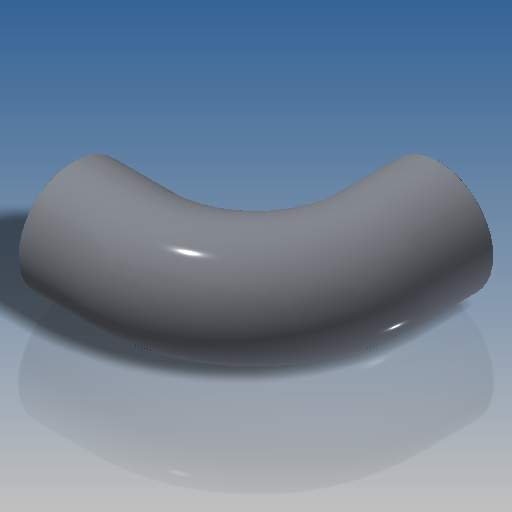
# Autodesk Inventor part: 25214-LtBluishGray
Saved by Autodesk Inventor 2019.4 (Build 234330000, 330)
## iProperties
Created: 2016-10-12
Part Number: 25214-LtBluishGray
Material: ABS Plastic
Document SubType Name: Modeling
Designer: D. Kohfeld
Density: 1.06 g/cm^3
Appearance: LtBluishGray
Mass: 0.6342 g
Surface Area: 8.19784 cm^2
Volume: 0.598302 cm^3
Author: D. Kohfeld
Autodesk Inventor part; units mm, degrees
ref_plane "YZ Plane" through (0, 0, 0) normal (1, 0, 0) x (0, 1, 0)
ref_plane "XZ Plane" through (0, 0, 0) normal (0, 1, 0) x (-1, 0, 0)
sketch "Sketch2" plane through (0, 0, 0) normal (0, 1, 0) x (-1, 0, 0)
  line L0 (0, -12) -> (0, -8)
  arc A0 (8, 0) -> (0, -8) centre (8, -8) ccw
  line L1 (8, 0) -> (12, 0)
  point P0 (0, 0)
  dimension "d0" = 4
  dimension "d1" = 8
  constraints: 4 end point, 2 point on circle, 2 tangent, 1 centre point, 1 horizontal, 1 horizontal alignment, 1 perpendicular, 1 vertical, 1 vertical alignment
  measures "d0" distance of L0.start L0.end
  measures "d1" radius of A0
ref_plane "Work Plane1" through (-12, 0, 0) normal (-1, 0, 0) x (0, -1, 0)
sketch "Sketch3" plane through (-12, 0, 0) normal (-1, 0, 0) x (0, -1, 0)
  circle A0 centre (0, 0) radius 3.6
  circle A1 centre (0, 0) radius 2.4
  line L0 (-2.2627, 0.8) -> (-1.6217, 0.8)
  arc A2 (-1.6217, 0.8) -> (-0.9998, 0.9998) centre (-1.6217, 1.8675) ccw
  line L1 (-0.8, 2.2627) -> (-0.8, 1.6217)
  arc A3 (-0.9998, 0.9998) -> (-0.8, 1.6217) centre (-1.8675, 1.6217) ccw
  line L2 (2.2627, -0.8) -> (1.6217, -0.8)
  arc A4 (1.6217, -0.8) -> (0.9998, -0.9998) centre (1.6217, -1.8675) ccw
  line L3 (0.8, -2.2627) -> (0.8, -1.6217)
  arc A5 (0.9998, -0.9998) -> (0.8, -1.6217) centre (1.8675, -1.6217) ccw
  line L4 (0.9998, -0.9998) -> (-0.9998, 0.9998) construction
  line L5 (-2.1108, -1.1421) -> (-1, -1)
  line L6 (-1, -1) -> (-1.1421, -2.1108)
  line L7 (2.1108, 1.1421) -> (1, 1)
  line L8 (1, 1) -> (1.1421, 2.1108)
  line L9 (-1, -1) -> (1, 1) construction
  point P0 (0, 0)
  dimension "d3" = 4.8
  dimension "d2" = 7.2
  dimension "d4" = 45
  dimension "d5" = 1.6
  dimension "d6" = 0.641
  dimension "d7" = 2.828
  dimension "d8" = 2
  dimension "d9" = 1.37
  constraints: 20 end point, 8 point on circle, 6 equal length, 5 centre point, 4 tangent, 3 coincident, 3 equal radius, 2 horizontal, 2 midpoint, 2 vertical, 1 perpendicular, 10 other
  measures "d2" diameter of A0
  measures "d4" angle of L3 L4
  measures "d5" distance between parallel lines of L2 L0
  measures "d6" distance of L1.start L1.end
  measures "d7" distance of L4.end L4.start
  measures "d8" horizontal distance of L5.end L7.end
  measures "d9" distance of L6.end L5.start
sweep "Sweep1" add profiles "Sketch3" path "Sketch2" contours A0 | A1 L2 A4 A5 L3 L6 L5 L0 A2 A3 L1 L8 L7 | L7 L8 A1 | A1 L3 A5 A4 L2 | L1 A3 A2 L0 A1 | A1 L5 L6
extrude "Extrusion1" cut sketch "Sketch3" against normal blind 8 contours A1 L2 A4 A5 L3 L6 L5 L0 A2 A3 L1 L8 L7
extrude "Extrusion2" cut sketch "Sketch3" against normal blind 1.6 contours L7 L8 A1 | A1 L3 A5 A4 L2 | L1 A3 A2 L0 A1 | A1 L5 L6
pattern_circular "Circular Pattern1" count 2 over 90 about axis through (0, -10, 0) along (0, -1, 0) of "Extrusion1", "Extrusion2"
fillet "Fillet1" radius 0.1 2 edges at (-12, 3.6, 0) (0, 3.6, -12)
equation "\"d0\" = 0.5 * lu"
equation "\"d1\" = lu"
equation "\"d3\" = kd"
equation "\"d2\" = tlad"
equation "\"d5\" = axlet"
equation "\"d12\" = lu"
equation "\"d14\" = wall"
equation "\"d19\" = lf"
equation "\"lu\" = 8"
equation "\"kd\" = 4.8"
equation "\"tlad\" = 7.2"
equation "\"axlet\" = 1.6"
equation "\"wall\" = 1.6"
equation "\"lf\" = 0.1"
body "Solid1"
